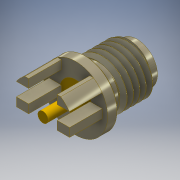
# Autodesk Inventor part: SMA Female Edge Mount CONSMA003-062
Saved by Autodesk Inventor 2016 (Build 200138000, 138)
## iProperties
Created: 2016-05-18
Part Number: SMA Female Edge Mount CONSMA003-062
Material: Generic
Document SubType Name: Modeling
Designer: Jonathan
Density: 1 g/cm^3
Appearance: Gold
Author: Jonathan
Autodesk Inventor part; units mm, degrees
ref_plane "YZ Plane" through (0, 0, 0) normal (1, 0, 0) x (0, 1, 0)
ref_plane "XZ Plane" through (0, 0, 0) normal (0, 1, 0) x (-1, 0, 0)
sketch "Sketch2" plane through (0, 0, 0) normal (0, 1, 0) x (-1, 0, 0)
  circle A0 centre (0, 0) radius 3.965
  dimension "d0" = 7.93
  constraints: 1 centre point, 1 coincident
  measures "d0" diameter of A0
extrude "Extrusion1" add sketch "Sketch2" along normal blind 1.26
sketch "Sketch4" plane through (0, 1.26, 0) normal (0, 1, 0) x (1, 0, 0)
  circle A0 centre (0, 0) radius 2.54
  dimension "d6" = 5.08
  constraints: 1 centre point, 1 coincident
  measures "d6" diameter of A0
extrude "Extrusion3" add sketch "Sketch4" along normal blind 6.35
sketch "Sketch5" plane through (0, 7.61, 0) normal (0, 1, 0) x (1, 0, 0)
  circle A0 centre (0, 0) radius 2.2987
  dimension "d9" = 4.5974
  constraints: 1 centre point, 1 coincident
  measures "d9" diameter of A0
extrude "Extrusion4" cut sketch "Sketch5" against normal blind 1.9304
sketch "Sketch6" plane through (0, 5.6796, 0) normal (0, 1, 0) x (1, 0, 0)
  circle A0 centre (0, 0) radius 2
  dimension "d12" = 4
  constraints: 1 centre point, 1 coincident
  measures "d12" diameter of A0
extrude "Extrusion5" cut sketch "Sketch6" against normal through all
sketch "Sketch7" plane through (0, 0, 0) normal (0, 1, 0) x (-1, 0, 0)
  circle A0 centre (0, 0) radius 2 projected
  circle A1 centre (0, 0) radius 0.635
  dimension "d15" = 1.27
  constraints: 1 centre point, 1 coincident
  measures "d15" diameter of A1
extrude "Extrusion6" add sketch "Sketch7" along normal up to surface (5.6796 mm away) separate body
sketch "Sketch8" plane through (0, 0, 0) normal (0, -1, 0) x (1, 0, 0)
  circle A0 centre (0, 0) radius 0.635 projected
extrude "Extrusion7" add sketch "Sketch8" against normal up to surface (5.6796 mm away) separate body
sketch "Sketch9" plane through (0, 5.6796, 0) normal (0, 1, 0) x (1, 0, 0)
  point P0 (0, 0)
  point P1 (0, 0)
  constraints: 1 coincident
hole "Hole2" at (0, 5.6796, 0) direction (0, -1, 0) diameter 1 depth 2.921 tip angle 118 bodies 3
sketch "Sketch10" plane through (0, 0, 0) normal (0, -1, 0) x (1, 0, 0)
  circle A0 centre (0, 0) radius 0.635 projected
  line L0 (3.302, 0.5334) -> (1.778, 0.5334)
  line L1 (1.778, 0.5334) -> (1.778, -0.5334)
  line L2 (1.778, -0.5334) -> (3.302, -0.5334)
  line L3 (3.302, -0.5334) -> (3.302, 0.5334)
  line L4 (3.302, 0.5334) -> (1.778, -0.5334) construction
  line L5 (1.778, 0.5334) -> (3.302, -0.5334) construction
  line L6 (-1.778, 0.5334) -> (-3.302, 0.5334)
  line L7 (-3.302, 0.5334) -> (-3.302, -0.5334)
  line L8 (-3.302, -0.5334) -> (-1.778, -0.5334)
  line L9 (-1.778, -0.5334) -> (-1.778, 0.5334)
  line L10 (-1.778, 0.5334) -> (-3.302, -0.5334) construction
  line L11 (-3.302, 0.5334) -> (-1.778, -0.5334) construction
  line L12 (1.7521, 3.3002) -> (1.7521, 2.2334)
  line L13 (1.7521, 2.2334) -> (3.2761, 2.2334)
  line L14 (3.376, 3.2955) -> (1.7521, 2.2334) construction
  line L15 (1.7521, 3.3002) -> (3.2761, 2.2334) construction
  line L16 (1.7521, 3.3002) -> (2.2015, 3.3002)
  circle A1 centre (0, 0) radius 0.635 projected
  circle A2 centre (0, 0) radius 3.965 projected
  line L17 (-1.778, 3.2618) -> (-1.778, 2.195)
  line L18 (-1.778, 2.195) -> (-3.302, 2.195)
  line L19 (-2.511, 2.7487) -> (-1.778, 2.195) construction
  line L20 (-1.778, 3.2618) -> (-3.302, 2.195) construction
  line L21 (-1.778, 3.2618) -> (-2.2543, 3.2618)
  arc A3 (3.2761, 2.2334) -> (2.1977, 3.3002) centre (0, 0) ccw
  arc A4 (-2.2543, 3.2618) -> (-3.302, 2.195) centre (0, 0) ccw
  point P0 (2.54, 0)
  point P1 (-2.54, 0)
  point P2 (2.54, 0)
  point P3 (2.54, 0)
  point P4 (-2.54, 0)
  point P5 (2.54, 2.7487)
  point P6 (2.5141, 2.7668)
  point P7 (2.5641, 2.7645)
  point P8 (-2.511, 2.7487)
  point P9 (-2.54, 0)
  point P10 (-2.54, 2.7284)
  dimension "d36" = 1.524
  dimension "d37" = 1.524
  dimension "d38" = 5.08
  dimension "d39" = 1.0668
  dimension "d40" = 1.0668
  dimension "d41" = 2.54
  dimension "d42" = 1.524
  dimension "d43" = 1.0668
  dimension "d44" = 1.7
  dimension "d45" = 1.0668
  dimension "d46" = 0.4494
  dimension "d51" = 1.524
  dimension "d53" = 1.0668
  constraints: 44 end point, 11 midpoint, 7 point on circle, 5 parallel, 5 point on line, 4 horizontal, 4 perpendicular, 3 horizontal alignment, 2 centre point, 2 coincident, 2 vertical alignment
  measures "d36" distance of L1.end L2.end
  measures "d37" distance of L7.end L8.end
  measures "d38" distance of point (-2.54, 0) point (2.54, 0)
  measures "d39" distance of L2.end L0.start
  measures "d40" distance of L6.end L7.end
  measures "d41" distance of point (0, 0) point (2.54, 0)
  measures "d42" distance of L12.end L13.end
  measures "d43" distance of L13.end L14.start
  measures "d44" distance between parallel lines of L13 L0
  measures "d45" distance of L12.start L12.end
  measures "d46" distance of L12.start L16.end
  measures "d51" distance of L17.end L18.end
  measures "d53" distance of L17.start L17.end
extrude "Extrusion8" add sketch "Sketch10" along normal blind 4.064 contours A0 | L3 L2 L1 L0 | L9 L8 L7 L6 | L16 A2 L13 L12 | L21 L17 L18 A2 bodies 2
sketch "Sketch11" plane through (0, 0, 0) normal (0, 0, 1) x (1, 0, 0)
  line L0 (-3.1009, 2.1417) -> (-2.54, 2.4656)
  line L1 (-2.54, 1.26) -> (-2.54, 7.61) projected
  line L2 (-2.54, 1.76) -> (-3.1009, 2.0838)
  line L3 (-2.54, 1.26) -> (2.54, 1.26) projected
  line L4 (-3.1009, 2.0838) -> (-3.1009, 2.1417)
  point P0 (0, 0)
  dimension "d60" = 0.5
  dimension "d62" = 120
  dimension "d63" = 0.7056
  dimension "d64" = 0.0579
  constraints: 6 end point, 2 point on line, 1 equal length, 1 vertical
  measures "d60" distance from line of L3 L2.start
  measures "d62" angle of L1 L0
  measures "d63" distance of L2.start L0.end
  measures "d64" distance of L2.end L0.start
coil "Coil1" sketch "Sketch11" operation add axis through (0, -10, 0) along (0, 1, 0) pitch 0.7857 turns 7 hand right bodies 1
sketch "Sketch12" plane through (0, 1.26, 0) normal (0, 1, 0) x (1, 0, 0)
  circle A0 centre (0, 0) radius 2.54 projected
  circle A1 centre (0, 0) radius 3.5
  dimension "d73" = 7
  constraints: 1 centre point, 1 coincident
  measures "d73" diameter of A1
extrude "Extrusion9" cut sketch "Sketch12" along normal blind 1.5 bodies 1
sketch "Sketch13" plane through (0, 7.61, 0) normal (0, 1, 0) x (1, 0, 0)
  circle A0 centre (0, 0) radius 5.7461
  arc A1 (-2.54, 0) -> (2.4278, 0.7465) centre (0, 0) ccw projected
  arc A2 (2.4278, 0.7465) -> (-2.54, 0) centre (0, 0) ccw projected
  dimension "d76" = 11.4922
  constraints: 1 centre point, 1 coincident
  measures "d76" diameter of A0
extrude "Extrusion10" cut sketch "Sketch13" along normal blind 1.5 and the other way blind 0.8 bodies 1
ref_plane "Work Plane1" through (2.54, 1.26, 0) normal (1, 0, 0) x (0, 1, 0)
sketch "Sketch14" plane through (2.54, 1.26, 0) normal (1, 0, 0) x (0, 1, 0)
  circle A0 centre (0.5, 0) radius 0.2286
  line L0 (0, 2.54) -> (0, -2.54) projected
  line L1 (-7.6588, 0) -> (8.6848, 0) projected
  line L2 (1.5, 2.5141) -> (1.5, 1.7989) projected
  line L3 (5.55, -0.4649) -> (5.55, 1.1207) projected
  line L4 (6.35, -2.54) -> (6.35, 2.54) projected
  line L5 (0, 2.54) -> (0, -2.54) projected
  point P0 (-1.26, 0)
  dimension "d81" = 0.4572
  dimension "d82" = 0.5
  constraints: 1 centre point, 1 point on line, 2 other
  measures "d81" diameter of A0
  measures "d82" distance from line of L0 A0.centre
extrude "Extrusion12" cut sketch "Sketch14" against normal blind 0.25 bodies 1
chamfer "Chamfer4" distance 0.05 angle 45 2 edges at (2.5297, 1.7601, 0.2286) (2.5297, 1.76, -0.2286)
pattern_circular "Circular Pattern1" count 4 over 360 about axis through (0, 1.26, 0) along (0, 1, 0) of "Extrusion12", "Chamfer4" bodies 1
chamfer "Chamfer3" distance 0.1 angle 45 2 edges at (3.965, 1.26, 0) (0, 5.6796, -0.5)
equation "\"d13\" = d12"
equation "\"d18\" = d12"
body "Solid1"
body "Solid2"
body "Solid3"
